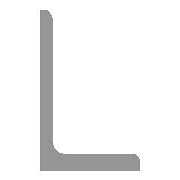
# Autodesk Inventor part: ANSI L 3 x 2 x 3_16 00000002
Saved by Autodesk Inventor 2021 (Build 250183000, 183)
## iProperties
Created: 2008-01-07
Part Number: ANSI L 3 x 2 x 3_16 00000002
Material: Generic
Document SubType Name: Modeling
Standard: AISC
Designer: nino.caldarola
Size Designation: L 3 x 2 x 3/16
Stock Number: L 3 x 2 x 3/16
Density: 1 g/cm^3
Description: Angle Steel
Standards Organization: ANSI
Language: en-US
Categories: <MemberInstance><Categories><Category DisplayName="Structural Shapes" InternalName="089c4875-fa83-4c05-b084-43b9cc11f5ed" Mnemonic="GRDR"><CategoryParameter DisplayName="Custom Base Point" InternalName="4f1d1b73-316d-484b-a3df-9cbabb16eb77" Mnemonic="shpBasePoint"/><CategoryParameter DisplayName="FG Authored" InternalName="9c666724-f362-4ea7-ac62-f6a007de5c69" Mnemonic="shpFGAuto"/><CategoryParameter DisplayName="Legacy Member ID" InternalName="340afe4f-75d7-48d3-ab7d-943f3c3da468" Mnemonic="LegacyMemberID"/><CategoryParameter DisplayName="Base Length" InternalName="42e34263-8f20-4d0e-ad48-bf1385b87c24" Mnemonic="shplen"/><CategoryParameter DisplayName="Distance of the Center of Gravity X-X" InternalName="26c9bdb8-9c79-4b4f-a92e-8e197583c9c4" Mnemonic="grcendistX"/><CategoryParameter DisplayName="Distance of the Center of Gravity Y-Y" InternalName="bcc4fb17-7af4-436a-8f8c-d0aa3b0248c5" Mnemonic="grcendistY"/><CategoryParameter DisplayName="Torsional Rigidity Modulus" InternalName="26c1ec35-5026-4c63-ad0a-751cf684a536" Mnemonic="torrigmod"/><CategoryParameter DisplayName="Torsional Section Modulus" InternalName="7c55a8dc-8844-49f9-a867-cc677b30ec9a" Mnemonic="torsecmod"/><CategoryParameter DisplayName="Coefficient of Shear Displacement" InternalName="de4c90c6-aaa8-468f-a335-6737b311b5d3" Mnemonic="shdispc"/><CategoryParameter DisplayName="Section Area" InternalName="1ff91680-64b0-4202-b9a3-7fd3f94bba3b" Mnemonic="secarea"/><CategoryParameter DisplayName="Moment of Inertia (x)" InternalName="4cd780bc-73d7-43ac-917a-579e5cbd684d" Mnemonic="inermomx"/><CategoryParameter DisplayName="Moment of Inertia (y)" InternalName="4b9f58ea-bced-460e-81ea-3d29ca5a49e3" Mnemonic="inermomy"/><CategoryParameter DisplayName="Section Module (x)" InternalName="72cfad18-cf51-4ed4-aaa7-c6b224f8419f" Mnemonic="secmodx"/><CategoryParameter DisplayName="Section Module (y)" InternalName="59eaa5e9-d227-48dc-b6c1-6920f96e0f95" Mnemonic="secmody"/><CategoryParameter DisplayName="Radius of Gyration (x)" InternalName="25778675-03e9-40c1-b6a8-4a9ed693320d" Mnemonic="gyrradx"/><CategoryParameter DisplayName="Radius of Gyration (y)" InternalName="bfa18ebe-1636-4dbe-8d42-b263e0b73184" Mnemonic="gyrrady"/><CategoryParameter DisplayName="Shape Thickness" InternalName="d109cf76-8eb4-42fc-9800-4409734adc67" Mnemonic="shpthick"/><CategoryParameter DisplayName="Second Shape Thickness" InternalName="9251a8e1-85fd-4e47-af99-afdb762317d9" Mnemonic="shpthick2"/><CategoryParameter DisplayName="Shape Width" InternalName="7c717d54-a18f-4666-b4d4-573cce22c62c" Mnemonic="shpwdth"/><CategoryParameter DisplayName="Shape Height" InternalName="50274e7d-5ac0-4796-92cb-c59e54983c67" Mnemonic="shpheig"/><CategoryParameter DisplayName="Mass per Length Unit" InternalName="0bb95a10-148f-4027-a459-38d7b056702a" Mnemonic="shpmass"/><CategoryParameter DisplayName="Section Designation" InternalName="5a64d034-428d-49c8-ba32-7619764de20f" Mnemonic="shpdes"/><Category DisplayName="Angles" InternalName="891838e5-6de8-44c9-8a56-cff30cd12e44" Mnemonic="LSHP"><CategoryParameter DisplayName="Moment of Inertia (x)" InternalName="fd23d820-fefc-47f1-b446-d1304eae789f" Mnemonic="inermomx"/><CategoryParameter DisplayName="Moment of Inertia (y)" InternalName="d0ed951c-e239-4172-87dd-dbe52d4ee0b6" Mnemonic="inermomy"/><CategoryParameter DisplayName="Section Module (x)" InternalName="e378446f-bf2e-4d99-93b0-32dd66c7caa2" Mnemonic="secmodx"/><CategoryParameter DisplayName="Section Module (y)" InternalName="efaf05a1-c4f1-4600-8633-7301da83f3ff" Mnemonic="secmody"/><CategoryParameter DisplayName="Section Area" InternalName="564a19c2-3cdb-4e61-a3cd-9a0c83be571a" Mnemonic="secarea"/><CategoryParameter DisplayName="Radius of Gyration (x)" InternalName="c9deb76c-754a-4e8e-9bc3-4870de9dfe62" Mnemonic="gyrradx"/><CategoryParameter DisplayName="Radius of Gyration (y)" InternalName="ff3a8a0d-cdc0-4094-bc22-17f67dad5d84" Mnemonic="gyrrady"/><CategoryParameter DisplayName="Shape Width" InternalName="22dbc2a2-e4da-47b4-bbc2-0ed25b88a7c5" Mnemonic="shpwdth"/><CategoryParameter DisplayName="Shape Thickness" InternalName="5c12cced-d35f-46db-9d8b-cf5f216ed4b9" Mnemonic="shpthick"/><CategoryParameter DisplayName="Second Shape Thickness" InternalName="e2df6b7d-3313-4ea2-80df-fc9eacf16587" Mnemonic="shpthick2"/><CategoryParameter DisplayName="Mass per Length Unit" InternalName="c045a850-bfad-4bdf-b14c-077eb4749b94" Mnemonic="shpmass"/></Category></Category></Categories><FamilyTemplate Id="gp0401in"><FamilyTemplateParameters><FamilyTemplateParameter ObjectType="kUserParameterObject" ValueType="xs:double" Id="2" ObjectReferenceKey="G_ER"/><FamilyTemplateParameter ObjectType="kUserParameterObject" ValueType="xs:double" Id="3" ObjectReferenceKey="G_H"/><FamilyTemplateParameter ObjectType="kUserParameterObject" ValueType="xs:double" Id="4" ObjectReferenceKey="B_L"/><FamilyTemplateParameter ObjectType="kUserParameterObject" ValueType="xs:double" Id="7" ObjectReferenceKey="G_W"/><FamilyTemplateParameter ObjectType="kUserParameterObject" ValueType="xs:double" Id="8" ObjectReferenceKey="G_T"/><FamilyTemplateParameter ObjectType="kUserParameterObject" ValueType="xs:double" Id="9" ObjectReferenceKey="G_IR"/><FamilyTemplateParameter ObjectType="kUserParameterObject" ValueType="xs:double" Id="118" ObjectReferenceKey="MAS"/><FamilyTemplateParameter ObjectType="kPropertyObject" ValueType="xs:string" Id="100" ObjectReferenceKey="{32853F0F-3444-11d1-9E93-0060B03C1CA6}" SubObjectId="52"/><FamilyTemplateParameter ObjectType="kPropertyObject" ValueType="xs:string" Id="105" ObjectReferenceKey="{32853F0F-3444-11d1-9E93-0060B03C1CA6}" SubObjectId="5"/><FamilyTemplateParameter ObjectType="kPartComponentDefinitionObject" ValueType="xs:string" Id="110" SubObjectId="Material"/><FamilyTemplateParameter ObjectType="kPropertyObject" ValueType="xs:string" Id="112" ObjectReferenceKey="{32853F0F-3444-11d1-9E93-0060B03C1CA6}" SubObjectId="55"/><FamilyTemplateParameter ObjectType="kiPartTableColumnObject" ValueType="xs:string" Id="404" ObjectReferenceKey="FILENAME"/><FamilyTemplateParameter ObjectType="kiPartTableColumnObject" ValueType="xs:string" Id="405" ObjectReferenceKey="MEMBER_REVISION"/><FamilyTemplateParameter ObjectType="kiPartTableColumnObject" ValueType="xs:string" Id="406" ObjectReferenceKey="G_D"/><FamilyTemplateParameter ObjectType="kiPartTableColumnObject" ValueType="xs:string" Id="407" ObjectReferenceKey="RID"/><FamilyTemplateParameter ObjectType="kiPartTableColumnObject" ValueType="xs:string" Id="408" ObjectReferenceKey="DACOOKIE"/></FamilyTemplateParameters></FamilyTemplate><CategoryParameterMap><ParamToTemplateMap><ParamToTemplate CategoryParameter="//CategoryParameter[@InternalName='9c666724-f362-4ea7-ac62-f6a007de5c69']" ConstantValue="1"/><ParamToTemplate CategoryParameter="//CategoryParameter[@InternalName='42e34263-8f20-4d0e-ad48-bf1385b87c24']" TemplateParameter="4"/><ParamToTemplate CategoryParameter="//CategoryParameter[@InternalName='316934ee-8fe1-4c7a-9c36-f2d79e1add1a']" TemplateParameter="408"/><ParamToTemplate CategoryParameter="//CategoryParameter[@InternalName='2675968c-4ce5-49e0-a4f5-552d29089031']" TemplateParameter="100"/><ParamToTemplate CategoryParameter="//CategoryParameter[@InternalName='8b46a4cc-9585-4fed-90c3-899f57e09a73']" TemplateParameter="404"/><ParamToTemplate CategoryParameter="//CategoryParameter[@InternalName='5a64d034-428d-49c8-ba32-7619764de20f']" TemplateParameter="406"/><ParamToTemplate CategoryParameter="//CategoryParameter[@InternalName='50274e7d-5ac0-4796-92cb-c59e54983c67']" TemplateParameter="3"/><ParamToTemplate CategoryParameter="//CategoryParameter[@InternalName='22dbc2a2-e4da-47b4-bbc2-0ed25b88a7c5']" TemplateParameter="7"/><ParamToTemplate CategoryParameter="//CategoryParameter[@InternalName='818a152a-d3c3-49ca-80ee-df7d91421b8e']" TemplateParameter="110"/><ParamToTemplate CategoryParameter="//CategoryParameter[@InternalName='a65d44b9-392f-4f4f-857b-e4b3d54996fe']" TemplateParameter="405"/><ParamToTemplate CategoryParameter="//CategoryParameter[@InternalName='016b6077-bfbe-49bd-92c9-d8d59c39c941']" TemplateParameter="105"/><ParamToTemplate CategoryParameter="//CategoryParameter[@InternalName='8e5e0294-fc51-4c8f-b3d7-003dc5ed94f6']" TemplateParameter="407"/><ParamToTemplate CategoryParameter="//CategoryParameter[@InternalName='4dba7c1c-e26c-444e-836c-b08b433409a8']" TemplateParameter="112"/></ParamToTemplateMap></CategoryParameterMap></MemberInstance>
Mass: 190.585 g
Surface Area: 813.214 cm^2
Volume: 190.585 cm^3
Appearance: Default
IsCustomPart: 1
_Version: 25.0.0
_CCFamilyMember: 5
_CCFamilyDisplayName: ANSI L (Unequal angles) - Angle Steel
G_L: 13.910 in
G_W: 2.000 in
G_H: 3.000 in
+33C3FEB4-CA1C-4392-B7BF-35601C3DAA07+CUTDETAIL1: Miter 67.50 deg
+F332B63C-46EB-47D4-9B6C-DFB219A39144+CUTDETAIL2: Miter 67.50 deg
Author: nino.caldarola
Autodesk Inventor part; units mm, degrees
ref_plane "Start plane" through (0, 0, -10.521) normal (0, 0, 1) x (1, 0, 0)
ref_plane "End plane" through (0, 0, 342.7905) normal (0, 0, 1) x (1, 0, 0)
sketch "Sketch" plane through (0, 0, 0) normal (0, 0, 1) x (1, 0, 0)
  line L0 (0, 76.2) -> (0, 0)
  line L1 (0, 0) -> (50.8, 0)
  line L2 (50.8, 0) -> (50.8, 2.7625)
  line L3 (48.8, 4.7625) -> (12.6365, 4.7625)
  line L4 (4.7625, 12.6365) -> (4.7625, 74.2)
  line L5 (2.7625, 76.2) -> (0, 76.2)
  line L6 (-7.0414, 0) -> (21.5385, 0) construction
  line L7 (0, -8.0414) -> (0, 34.5385) construction
  arc A0 (4.7625, 12.6365) -> (12.6365, 4.7625) centre (12.6365, 12.6365) ccw
  arc A1 (50.8, 2.7625) -> (48.8, 4.7625) centre (48.8, 2.7625) ccw
  arc A2 (4.7625, 74.2) -> (2.7625, 76.2) centre (2.7625, 74.2) ccw
  line L8 (0, 93.5453) -> (0, -24.9725) construction
  line L9 (-18.6925, 0) -> (62.8653, 0) construction
  point P0 (50.8, 4.7625)
  point P1 (4.7625, 4.7625)
  point P2 (4.7625, 76.2)
  dimension "d12" = 4.7625
  dimension "d13" = 76.2
  dimension "d14" = 50.8
  dimension "d15" = 0
  dimension "d16" = 4.7625
  dimension "d17" = 0
  dimension "d18" = 7.874
  dimension "d19" = 2
  constraints: 16 end point, 6 point on circle, 6 point on line, 6 tangent, 3 centre point, 2 collinear, 2 parallel, 1 equal radius
  measures "d12" distance between parallel lines of L4 L0
  measures "d13" distance of L0.start L1.start
  measures "d14" distance of L1.start L1.end
  measures "d15" distance between parallel lines of L6 L1
  measures "d16" distance between parallel lines of L1 L3
  measures "d17" distance between parallel lines of L7 L0
  measures "d18" radius of A0
  measures "d19" radius of A1
extrude "Body" add sketch "Sketch" along normal up to surface (353.3115 mm away) from surface at -10.521
sketch "Sketch3" plane through (0, 0, 0) normal (0, 0, 1) x (1, 0, 0)
  line L0 (0, 0) -> (10, 0)
ref_plane "Work Plane5" through (0, 0, 0) normal (0, -1, 0) x (1, 0, 0)
sketch "Sketch4" plane through (0, 0, 0) normal (0, -1, 0) x (1, 0, 0)
  line L0 (-2, -10.521) -> (12, -10.521)
  line L1 (-2, 342.7905) -> (12, 342.7905)
  dimension "d23" = 353.3115
  measures "d23" distance between parallel lines of L0 L1
ref_plane "Work Plane3" through (50.8, 38.1, -10.521) normal (-0.3827, 0, -0.9239) x (-0.9239, 0, 0.3827)
split "Split1" plane through (50.8, 38.1, -10.521) removes the side toward (-0.3827, 0, -0.9239)
ref_plane "Work Plane4" through (50.8, 38.1, 342.7905) normal (-0.3827, 0, 0.9239) x (0.9239, 0, 0.3827)
split "Split2" plane through (50.8, 38.1, 342.7905) removes the side toward (-0.3827, 0, 0.9239)
equation "\"d12\" = G_T"
equation "\"d13\" = G_H"
equation "\"d14\" = G_W"
equation "\"d16\" = G_T"
equation "\"d18\" = G_IR"
equation "\"d4\" = G_L"
equation "\"G_W\" = 50.8"
equation "\"G_H\" = 76.2"
equation "\"G_T\" = 4.7625"
equation "\"G_ER\" = 4.064"
equation "\"G_IR\" = 7.874"
equation "\"G_L\" = d23"
equation "\"ex\" = 0"
equation "\"ey\" = 0"
equation "\"G_OFFSET_START\" = 10.52102"
equation "\"G_OFFSET_END\" = 10.52102"
equation "\"d20\" = -G_OFFSET_START"
equation "\"d21\" = G_OFFSET_END + B_L"
equation "\"B_L\" = 332.26948"
body "Solid1"
